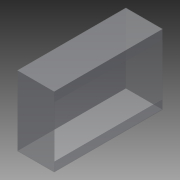
# Autodesk Inventor part: box_middlegoal
Saved by Autodesk Inventor 2013 (Build 170138000, 138)
## iProperties
Created: 2012-12-31
Part Number: box_middlegoal
Material: Polycarbonate, Clear
Document SubType Name: Modeling
Designer: Phillip
Density: 1 g/cm^3
Author: Phillip
Autodesk Inventor part; units mm, degrees
ref_plane "YZ Plane" through (0, 0, 0) normal (1, 0, 0) x (0, 1, 0)
ref_plane "XZ Plane" through (0, 0, 0) normal (0, 1, 0) x (-1, 0, 0)
ref_plane "XY Plane" through (0, 0, 0) normal (0, 0, 1) x (1, 0, 0)
sketch "Sketch1" plane through (0, 0, 0) normal (0, 0, 1) x (1, 0, 0)
  line L0 (-749.3, -254) -> (749.3, -254)
  line L1 (749.3, -254) -> (749.3, 254)
  line L2 (749.3, 254) -> (-749.3, 254)
  line L3 (-749.3, 254) -> (-749.3, -254)
  line L4 (-749.3, -254) -> (749.3, 254) construction
  line L5 (749.3, -254) -> (-749.3, 254) construction
  point P0 (0, 0)
  dimension "d0" = 1498.6
  dimension "d1" = 508
  constraints: 12 end point, 2 midpoint, 2 parallel, 1 horizontal, 1 perpendicular
  measures "d0" distance of L2.end L1.end
  measures "d1" distance of L1.end L0.end
extrude "Extrusion1" add sketch "Sketch1" against normal blind 965.2
shell "Shell1" thickness 3.175 removed faces 0
sketch "Sketch2" plane through (-749.3, -254, 0) normal (0, -1, 0) x (1, 0, 0)
  line L0 (0, 0) -> (1498.6, 0) projected
  line L1 (1498.6, -965.2) -> (0, -965.2) projected
  line L2 (3.175, -127) -> (1495.425, -127)
  line L3 (1495.425, -127) -> (1495.425, -838.2)
  line L4 (1495.425, -838.2) -> (3.175, -838.2)
  line L5 (3.175, -838.2) -> (3.175, -127)
  line L6 (3.175, -3.175) -> (3.175, -962.025) projected
  line L7 (1495.425, -3.175) -> (1495.425, -962.025) projected
  point P0 (749.3, 0)
  dimension "d5" = 127
  dimension "d6" = 127
  constraints: 8 end point, 2 collinear, 2 parallel, 1 horizontal, 1 perpendicular
  measures "d5" distance between parallel lines of L0 L2
  measures "d6" distance between parallel lines of L1 L4
extrude "Extrusion2" cut sketch "Sketch2" against normal blind 3.175
equation "\"d6\" = d5"
body "Solid1"
